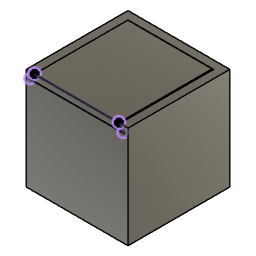
Slide top box v3 (Autodesk Fusion 360 design; units mm, degrees)
Autodesk Fusion 360 part; units mm, degrees
sketch "Sketch1" plane through (0, 0, 0) normal (0, 0, 1) x (1, 0, 0) in component "lid"
box "BoxPrimitive1" add length 50 width 50 height 50 placed x (0, 1, 0) y (-1, 0, 0) z (0, 0, 1) at (50, 0, 0) makes body 1 in component "BOX"
shell "Shell1" thickness 4 removed faces 1 at (16.6667, 16.6667, 50) on bodies 1 in component "BOX"
sketch "Sketch2" plane through (0, 0, 0) normal (0, -1, 0) x (1, 0, 0) in component "BOX"
  line L0 (0, 50) -> (0, 0)
  line L1 (0, 0) -> (50, 0)
  line L2 (50, 0) -> (50, 50)
  line L3 (50, 50) -> (0, 50)
  line L4 (46, 50) -> (48.2943, 46.7234)
  line L5 (46, 50) -> (50, 50) construction
  line L6 (25, 50) -> (25, 46.7234) construction
  line L7 (25, 46.7234) -> (48.2943, 46.7234)
  line L8 (25, 46.7234) -> (1.7057, 46.7234)
  line L9 (4, 50) -> (1.7057, 46.7234)
  dimension "d7" = 55
  dimension "d8" = 4
  constraint horizontal L5
  constraint coincident L3 L4.start
  constraint midpoint L3 L6.start
  constraint perpendicular L3 L6
  constraint horizontal L4.end L6.end
  constraint symmetric L4.start L6 L9.start
  constraint symmetric L4.end L6 L8.end
  constraint symmetric L7.start L6 L8.start
  measures "d7" angle of L4 L5
  measures "d8" distance of L4.start L4.end
extrude "Extrude1" cut sketch "Sketch2" against normal blind 46 contours L3 L4 L7 L8 L9 bodies 1 in component "BOX"
sketch "Sketch2 (2)" plane through (0, 0, 0) normal (0, -1, 0) x (1, 0, 0) in component "lid"
  line L0 (1.7057, 46.7234) -> (4, 50)
  line L1 (4, 50) -> (0, 50)
  line L2 (0, 50) -> (0, 0)
  line L3 (0, 0) -> (50, 0)
  line L4 (50, 0) -> (50, 50)
  line L5 (50, 50) -> (46, 50)
  line L6 (46, 50) -> (48.2943, 46.7234)
  line L7 (48.2943, 46.7234) -> (1.7057, 46.7234)
  line L8 (48.2943, 46.7234) -> (1.7057, 46.7234)
  line L9 (1.7057, 46.7234) -> (4, 50)
  line L10 (4, 50) -> (46, 50)
  line L11 (46, 50) -> (48.2943, 46.7234)
  line L12 (47.8141, 46.9734) -> (2.1859, 46.9734)
  line L13 (2.1859, 46.9734) -> (4.4802, 50.25)
  line L14 (4.4802, 50.25) -> (-0.25, 50.25)
  line L15 (-0.25, 50.25) -> (-0.25, -0.25)
  line L16 (-0.25, -0.25) -> (50.25, -0.25)
  line L17 (50.25, -0.25) -> (50.25, 50.25)
  line L18 (50.25, 50.25) -> (45.5198, 50.25)
  line L19 (45.5198, 50.25) -> (47.8141, 46.9734)
  dimension "d11" = 0.25
sketch "Sketch3" plane through (0, 0, 0) normal (0, -1, 0) x (1, 0, 0) in component "lid"
  line L0 (45.5198, 50.25) -> (47.8141, 46.9734)
  line L1 (4, 50) -> (46, 50)
  line L2 (2.1859, 46.9734) -> (4.4802, 50.25)
  line L3 (45.6948, 50) -> (4.3052, 50)
  constraint coincident L0 L3.start
  constraint coincident L1 L3.start
  constraint coincident L2 L3.end
  constraint coincident L1 L3.end
extrude "Extrude1'" add sketch "Sketch2 (2)" along normal blind 46 from surface at -45.75 separate body contours L10 L12 L13 L19 makes body 2 in component "lid"
component "BOX" placed x (1, 0, 0) y (0, 1, 0) z (0, 0, 1) at (0, 0, 0)
component "lid" placed x (1, 0, 0) y (0, 1, 0) z (0, 0, 1) at (-0.3927, 0.25, -0.125)
